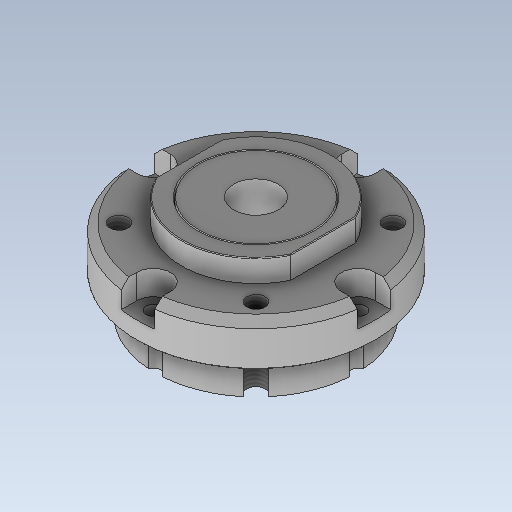
# Autodesk Inventor part: 555_GearBox_FrontCover
Saved by Autodesk Inventor 2021 (Build 250183000, 183)
## iProperties
Created: 2021-08-07
Part Number: 555_GearBox_FrontCover
Material: 一般
Document SubType Name: Modeling
Designer: Hagihara Yuya
Density: 1 g/cm^3
Appearance: 淡い灰色
Author: Hagihara Yuya
Autodesk Inventor part; units mm, degrees
ref_plane "YZ Plane" through (0, 0, 0) normal (1, 0, 0) x (0, 1, 0)
ref_plane "XZ Plane" through (0, 0, 0) normal (0, 1, 0) x (-1, 0, 0)
ref_plane "XY Plane" through (0, 0, 0) normal (0, 0, 1) x (1, 0, 0)
sketch "スケッチ1" plane through (0, 0, 0) normal (0, 0, 1) x (1, 0, 0)
  circle A0 centre (0, 0) radius 16
  dimension "d0" = 32
  constraints: 1 centre point, 1 coincident
  measures "d0" diameter of A0
extrude "押し出し1" add sketch "スケッチ1" along normal blind 5.7
sketch "スケッチ2" plane through (0, 0, 0) normal (0, 0, -1) x (-1, 0, 0)
  circle A0 centre (0, 0) radius 13.5
  dimension "d3" = 27
  constraints: 1 centre point, 1 coincident
  measures "d3" diameter of A0
extrude "押し出し2" add sketch "スケッチ2" along normal blind 5
sketch "スケッチ3" plane through (0, 0, 5.7) normal (0, 0, 1) x (1, 0, 0)
  circle A0 centre (0, 0) radius 10
  line L0 (-9, 4.3589) -> (9, 4.3589) construction
  line L1 (9, 4.3589) -> (9, -4.3589)
  line L2 (9, -4.3589) -> (-9, -4.3589) construction
  line L3 (-9, -4.3589) -> (-9, 4.3589)
  dimension "d6" = 20
  dimension "d7" = 18
  constraints: 8 end point, 3 point on circle, 2 parallel, 1 centre point, 1 coincident, 1 horizontal, 1 perpendicular
  measures "d6" diameter of A0
  measures "d7" distance of L0.start L0.end
extrude "押し出し3" add sketch "スケッチ3" along normal blind 3 contours L1 A0 L3
sketch "スケッチ4" plane through (0, 0, 8.7) normal (0, 0, 1) x (1, 0, 0)
  point P0 (0, 0)
  point P1 (0, 0)
  constraints: 1 coincident
hole "穴1" at (0, 0, 8.7) direction (0, 0, -1) diameter 6 end through all
sketch "スケッチ5" plane through (0, 0, 5.7) normal (0, 0, 1) x (1, 0, 0)
  circle A0 centre (0, 13.75) radius 2.25
  line L0 (-2.25, 13.75) -> (2.25, 13.75)
  line L1 (2.25, 13.75) -> (2.25, 16)
  line L2 (2.25, 16) -> (-2.25, 16)
  line L3 (-2.25, 16) -> (-2.25, 13.75)
  circle A1 centre (0, 0) radius 16 projected
  circle A2 centre (-13.75, 0) radius 2.25
  line L4 (-13.75, -2.25) -> (-13.75, 2.25)
  line L5 (-13.75, 2.25) -> (-16, 2.25)
  line L6 (-16, 2.25) -> (-16, -2.25)
  line L7 (-16, -2.25) -> (-13.75, -2.25)
  circle A3 centre (0, -13.75) radius 2.25
  line L8 (2.25, -13.75) -> (-2.25, -13.75)
  line L9 (-2.25, -13.75) -> (-2.25, -16)
  line L10 (-2.25, -16) -> (2.25, -16)
  line L11 (2.25, -16) -> (2.25, -13.75)
  circle A4 centre (13.75, 0) radius 2.25
  line L12 (13.75, 2.25) -> (13.75, -2.25)
  line L13 (13.75, -2.25) -> (16, -2.25)
  line L14 (16, -2.25) -> (16, 2.25)
  line L15 (16, 2.25) -> (13.75, 2.25)
  point P0 (-15.841, -2.25)
  point P1 (-15.841, 2.25)
  point P2 (2.25, -15.841)
  point P3 (-2.25, -15.841)
  point P4 (15.841, -2.25)
  point P5 (15.841, 2.25)
  point P6 (2.25, 15.841)
  point P7 (-2.25, 15.841)
  dimension "d17" = 4.5
  dimension "d18" = 13.75
  dimension "d21" = 360
  constraints: 32 end point, 8 point on circle, 4 centre point, 4 coincident, 2 parallel, 1 horizontal, 1 midpoint, 1 perpendicular, 1 tangent, 1 vertical alignment, 45 other
  measures "d17" diameter of A0
  measures "d18" distance of point (0, 0) A0.centre
extrude "押し出し4" cut sketch "スケッチ5" against normal blind 3.3 contours L0 A0 | L3 A1 A0 | A0 L0 | A0 A1 L1 | L5 A2 A1 | A1 A4 L15 | A2 L7 A1 | A2 L4 | A2 L4 | A4 L12 | A1 L13 A4 | L12 A4 | L9 A3 A1 | A1 A3 L11 | A3 L8 | A3 L8
sketch "スケッチ6" plane through (0, 0, 2.4) normal (0, 0, 1) x (1, 0, 0)
  arc A0 (-2.25, 13.75) -> (2.25, 13.75) centre (0, 13.75) ccw projected
  arc A1 (13.75, 2.25) -> (13.75, -2.25) centre (13.75, 0) ccw projected
  arc A2 (2.25, -13.75) -> (-2.25, -13.75) centre (0, -13.75) ccw projected
  arc A3 (-13.75, -2.25) -> (-13.75, 2.25) centre (-13.75, 0) ccw projected
  point P0 (0, 0)
  constraints: 4 coincident
hole "穴2" at (0, 13.75, 2.4) at (13.75, 0, 2.4) at (0, -13.75, 2.4) at (-13.75, 0, 2.4) direction (0, 0, -1) diameter 2 end through all
sketch "スケッチ7" plane through (0, 0, 5.7) normal (0, 0, 1) x (1, 0, 0)
  line L0 (9.1924, 9.1924) -> (0, 0) construction
  line L1 (-22.4, 0) -> (22.4, 0) projected
  point P0 (-9.1924, 9.1924)
  point P1 (-9.1924, -9.1924)
  point P2 (9.1924, -9.1924)
  dimension "d32" = 45
  dimension "d33" = 13
  dimension "d36" = 360
  constraints: 2 end point, 5 other
  measures "d32" angle of L1 L0
  measures "d33" distance of L0.start L0.end
hole "穴3" at (9.1924, 9.1924, 5.7) at (-9.1924, 9.1924, 5.7) at (-9.1924, -9.1924, 5.7) at (9.1924, -9.1924, 5.7) direction (0, 0, -1) diameter 2.459 end through all thread size "M3x0.5" class "6H" standard "ISO Metric profile"
sketch "スケッチ8" plane through (0, 0, 8.7) normal (0, 0, 1) x (1, 0, 0)
  circle A0 centre (0, 0) radius 3 projected
  circle A1 centre (0, 0) radius 7.65
  circle A2 centre (0, 0) radius 7.85
  dimension "d45" = 15.3
  dimension "d46" = 15.7
  constraints: 2 centre point, 2 coincident
  measures "d45" diameter of A1
  measures "d46" diameter of A2
extrude "押し出し5" cut sketch "スケッチ8" against normal up to surface (3 mm away) contours A2
chamfer "面取り1" distance 1 angle 45 4 edges at (11.3137, -11.3137, 5.7) (-11.3137, -11.3137, 5.7) (-11.3137, 11.3137, 5.7) (11.3137, 11.3137, 5.7)
fillet "フィレット1" radius 0.1 5 edges at (-16, 0, 0) (0, -10, 8.7) (9, 0, 8.7) (0, 10, 8.7) (-9, 0, 8.7)
